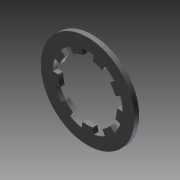
# Autodesk Inventor part: AT509
Saved by Autodesk Inventor 2015 (Build 190159000, 159)
## iProperties
Category: PARTsolutions
Company: NKKSWITCHES
Created: 2015-01-04
Part Number: AT509
Catalog Web Link: www.cadenas.de
Description: Lockwasher - Bushing Mount Miniature Toggles-Series M - Standard Hardwarw for Small & Large Bushings
Vendor: NKKSWITCHES
Document SubType Name: Modeling
Designer: PARTuser1
Manufacturer: NKKSWITCHES
Mass: 0.0218415 g
Surface Area: 1.19048 cm^2
Volume: 0.0218415 cm^3
Density: 1 g/cm^3
Material: Generic
Appearance: PSOLRGB-242-242-242
PSOL_IDENT_0: {$CADENAS_DATA\23d-libs\nkkswitches\toggle\m\hardware\lockwasher.prj},181 {VTYP=3D},{NB=AT509},{LINA=
PSOL_IDENT_1: AT509},{NN=Lockwasher - Bushing Mount Miniature Toggles},{DATE=21.11.2014 08:56:33},{GEOMDATE=11.10.
PSOL_IDENT_2: 2006},{VERSION=},{LINEID=10},{LINESUBID=-1},{WBVAR=}  {NB=AT509},{LINA=AT509},{KT=DUMMY},{PN=AT509},
PSOL_IDENT_3: {D=0.402},{DD=0.252},{T=0.020}
SUPPLIER: NKKSWITCHES
ARTICLENO: AT509
BOMINFO: AT509
CREATOR: CADENAS GmbH
Title: AT509
Author: Cadenas PARTsolutions
Comments: Series M - Standard Hardwarw for Small & Large Bushings
Autodesk Inventor part; units mm, degrees
sketch "Sketch_2" plane through (0, 0, 0) normal (0, 0, 1) x (1, 0, 0)
  circle A0 centre (0, 0) radius 5.1054
  line L0 (-3.81, 0) -> (-3.2004, 0)
  arc A1 (-3.2004, 0) -> (-3.0074, -1.0946) centre (0, 0) ccw
  line L1 (-3.0074, -1.0946) -> (-3.5802, -1.3031)
  arc A2 (-3.5802, -1.3031) -> (-2.9186, -2.449) centre (0, 0) ccw
  line L2 (-2.9186, -2.449) -> (-2.4516, -2.0572)
  arc A3 (-2.4516, -2.0572) -> (-1.6002, -2.7716) centre (0, 0) ccw
  line L3 (-1.6002, -2.7716) -> (-1.905, -3.2996)
  arc A4 (-1.905, -3.2996) -> (-0.6616, -3.7521) centre (0, 0) ccw
  line L4 (-0.6616, -3.7521) -> (-0.5557, -3.1518)
  arc A5 (-0.5557, -3.1518) -> (0.5557, -3.1518) centre (0, 0) ccw
  line L5 (0.5557, -3.1518) -> (0.6616, -3.7521)
  arc A6 (0.6616, -3.7521) -> (1.905, -3.2996) centre (0, 0) ccw
  line L6 (1.905, -3.2996) -> (1.6002, -2.7716)
  arc A7 (1.6002, -2.7716) -> (2.4516, -2.0572) centre (0, 0) ccw
  line L7 (2.4516, -2.0572) -> (2.9186, -2.449)
  arc A8 (2.9186, -2.449) -> (3.5802, -1.3031) centre (0, 0) ccw
  line L8 (3.5802, -1.3031) -> (3.0074, -1.0946)
  arc A9 (3.0074, -1.0946) -> (3.2004, 0) centre (0, 0) ccw
  line L9 (3.2004, 0) -> (3.81, 0)
  arc A10 (3.81, 0) -> (3.5802, 1.3031) centre (0, 0) ccw
  line L10 (3.5802, 1.3031) -> (3.0074, 1.0946)
  arc A11 (3.0074, 1.0946) -> (2.4516, 2.0572) centre (0, 0) ccw
  line L11 (2.4516, 2.0572) -> (2.9186, 2.449)
  arc A12 (2.9186, 2.449) -> (1.905, 3.2996) centre (0, 0) ccw
  line L12 (1.905, 3.2996) -> (1.6002, 2.7716)
  arc A13 (1.6002, 2.7716) -> (0.5557, 3.1518) centre (0, 0) ccw
  line L13 (0.5557, 3.1518) -> (0.6616, 3.7521)
  arc A14 (0.6616, 3.7521) -> (-0.6616, 3.7521) centre (0, 0) ccw
  line L14 (-0.6616, 3.7521) -> (-0.5557, 3.1518)
  arc A15 (-0.5557, 3.1518) -> (-1.6002, 2.7716) centre (0, 0) ccw
  line L15 (-1.6002, 2.7716) -> (-1.905, 3.2996)
  arc A16 (-1.905, 3.2996) -> (-2.9186, 2.449) centre (0, 0) ccw
  line L16 (-2.9186, 2.449) -> (-2.4516, 2.0572)
  arc A17 (-2.4516, 2.0572) -> (-3.0074, 1.0946) centre (0, 0) ccw
  line L17 (-3.0074, 1.0946) -> (-3.5802, 1.3031)
  arc A18 (-3.5802, 1.3031) -> (-3.81, 0) centre (0, 0) ccw
  constraints: 36 end point, 36 point on circle, 19 centre point
extrude "Extrusion1" add sketch "Sketch_2" along normal mid plane 0.508
ref_plane "lockwasher_XY" through (0, 0, 0.254) normal (0, 0, 1) x (1, 0, 0)
ref_plane "lockwasher_YZ" through (0, 0, 0.254) normal (1, 0, 0) x (0, 1, 0)
ref_plane "lockwasher_ZX" through (0, 0, 0.254) normal (0, 1, 0) x (0, 0, 1)
body "Solid1"
